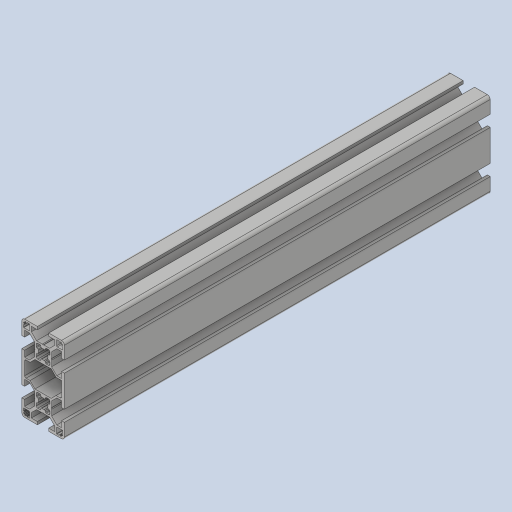
# Autodesk Inventor part: HFSLB6-3060-300
Saved by Autodesk Inventor 2023 (Build 270158000, 158)
## iProperties
Created: 2024-09-13
Part Number: HFSLB6-3060-300
Material: Generic
Catalog Web Link: www.cadenas.de
Description: NEFS6-3060, NEFSB6-3060, NEFSY6-3060, EFS6-3060, EFSB6-3060, HFS6-3060, HFSB6-3060, CAF6-3060, NFSL6-3060, HFSL6-3060, HFSLB6-3060, GFS6-3060, HFSY6-3060-Aluminum Frames -6 Series-2 Row Groove 30x60 mm Square-Specified Length
Vendor: MISUMI
Document SubType Name: Modeling
Designer: psAdmin
Manufacturer: MISUMI
Mass: 145.426 g
Surface Area: 1809.35 cm^2
Volume: 145.426 cm^3
Density: 1 g/cm^3
Appearance: PSOLRGB-175-175-175
Category: PARTsolutions
Company: MISUMI
PSOL_IDENT_0: {$CADENAS_DATA/23d-libs/misumi/metric/38_al_extrusions_blackets/6/hfs6_3060.prj},759 {VTYP=3D},{NB=H
PSOL_IDENT_1: FSLB6-3060-300},{LINA=HFSLB6-3060-300},{NN=NEFS6-3060, NEFSB6-3060, NEFSY6-3060, EFS6-3060, EFSB6-30
PSOL_IDENT_2: 60, HFS6-3060, HFSB6-3060, CAF6-3060, NFSL6-3060, HFSL6-3060, HFSLB6-3060, GFS6-3060, HFSY6-3060},{D
PSOL_IDENT_3: ATE=31.01.2024 10:05:17},{GEOMDATE=26.07.2023 02:49:00},{VERSION=},{LINEID=70},{WBVAR=L,ALT1,ALT2,AL
PSOL_IDENT_4: T3,ALT4,ALT5,CP5,DL5,DR5,ALT6,ALT9,ALT10,ALT11,DD6SE,DD6,HP6,NHL6,DL6,NHR6,DR6,ALT7,ALT8,NH9,AH,BH,C
PSOL_IDENT_5: H,DH,EH,NH10,AV,BV,CV,DV,EV,NH11,AP,BP,CP,DP,EP,ALT12,ALT13,Z,NH12,XA,XB,XC,XD,XE,NH13,YA,YB,YC,YD,Y
PSOL_IDENT_6: E,ALT14,HP14,DL14,DR14,ALT15,HP15,DL15,DR15,ALT16,HP16,DL16,DR16,ALT17,HQ17,JLP,ALT18,HQ18,KLP,ALT19
PSOL_IDENT_7: ,ALT20},{WBNUMERIC=L,DD6,NH9,AH,BH,CH,DH,EH,NH10,AV,BV,CV,DV,EV,NH11,AP,BP,CP,DP,EP,NH12,XA,XB,XC,XD
PSOL_IDENT_8: ,XE,NH13,YA,YB,YC,YD,YE,HQ17,JLP,HQ18,KLP}  {NB=HFSLB6-3060-300},{LINA=HFSLB6-3060-300},{KT=DUMMY},{
PSOL_IDENT_9: PN=HFSLB6-3060-300},{TPS=HFSLB6-3060},{MAT=A6N01SS-T5 Aluminum Alloy},{ST=Black Anodize},{FRMW=30},{
PSOL_IDENT_10: FRMH=60},{FRD=6.8},{L=300.0},{MASS=1.29},{SA=476},{LX=4.87x10^4},{LY=17.87x10^4},{ALT1=},{M1=0},{IDM
PSOL_IDENT_11: 1=6.647},{DALT1=4.2},{DPL1=0},{DPR1=0},{ALT1PN=},{ALT2=},{ALT2ALG= '','w/o End Tapping (Insert)','LH
PSOL_IDENT_12: P','with LHP (Tapping on the Left (Insert))','RHP','with RHP (Tapping on the Right (Insert))','HPW','
PSOL_IDENT_13: with HPW (Tapping on Both Ends (Insert))' },{M2=0},{DP2=0},{ALT2PN=},{ALT3=},{ALT3ALG= '','N/A' },{M
PSOL_IDENT_14: 3=0},{IDM3=4.134},{DP3=0},{ALT3PN=},{ALT4=},{ALT4ALG= '', 'w/o SC (High Precision Cut)', 'SC', 'with
PSOL_IDENT_15: SC (High Precision Cut)' },{ALT4PN=},{ALT5=},{ALT5ALG= '','w/o 45 Degree Cut','1','with 45 Degree C
PSOL_IDENT_16: ut' },{CP5=},{CP5ALG= '','N/A' },{DL5=},{DL5ALG= '','N/A' },{DR5=},{DR5ALG= '','N/A' },{FRMLALT5=0},
PSOL_IDENT_17: {FRMRALT5=0},{ALT5PN=},{ALT6=},{ALT6ALG= '','w/o Fastening Location Wrench Access Hole Alterations','
PSOL_IDENT_18: 1','with Fastening Location Wrench Access Hole Alterations' },{ALT9=},{ALT9ALG= '','w/o Location Spe
PSOL_IDENT_19: cified Wrench Access Hole Alteratons (Horizontal)','1','with Location Specified Wrench Access Hole A
PSOL_IDENT_20: lteratons (Horizontal)' },{ALT10=},{ALT10ALG= '','w/o Location Specified Wrench Access Hole Alterato
PSOL_IDENT_21: ns (Vertical)','1','with Location Specified Wrench Access Hole Alteratons (Vertical)' },{ALT11=},{AL
PSOL_IDENT_22: T11ALG= '','w/o Location Specified Wrench Access Hole Alteratons (Crisscross)','1','with Location Sp
PSOL_IDENT_23: ecified Wrench Access Hole Alteratons (Crisscross)' },{DD6SE=},{DD6SEALG= '','N/A' },{DD6=0},{DD6ALG=
PSOL_IDENT_24: 0},{HP6=},{HP6ALG= '','N/A' },{NHL6=},{NHL6ALG= '','N/A' },{DL6=},{DL6ALG= '','N/A' },{NHR6=},{NHR6A
PSOL_IDENT_25: LG= '','N/A' },{DR6=},{DR6ALG= '','N/A' },{DD6PN=},{HL6=0},{HL6D=0},{HR6=0},{HR6D=0},{J6=0},{J6D=0},
PSOL_IDENT_26: {K6=0},{K6D=0},{ALT7=},{ALT7ALG= '','N/A' },{ALT8=},{ALT8ALG= '','N/A' },{ALT678PN=},{NH9=0},{NH9MAX=
PSOL_IDENT_27: 5},{NH9ALG=[0]},{AH=0.0},{AHMIN=7},{AHMAX=295},{AHALG=[0]},{BH=0.0},{BHMIN=2},{BHMAX=297},{BHALG=[0]
PSOL_IDENT_28: },{CH=0.0},{CHMIN=2},{CHMAX=299},{CHALG=[0]},{DH=0.0},{DHMIN=2},{DHMAX=301},{DHALG=[0]},{EH=0.0},{EH
PSOL_IDENT_29: MIN=2},{EHMAX=293},{EHALG=[0]},{NH10=0},{NH10MAX=5},{NH10ALG=[0]},{AV=0.0},{AVMIN=7},{AVMAX=295},{AV
PSOL_IDENT_30: ALG=[0]},{BV=0.0},{BVMIN=2},{BVMAX=297},{BVALG=[0]},{CV=0.0},{CVMIN=2},{CVMAX=299},{CVALG=[0]},{DV=0
PSOL_IDENT_31: .0},{DVMIN=2},{DVMAX=301},{DVALG=[0]},{EV=0.0},{EVMIN=2},{EVMAX=293},{EVALG=[0]},{NH11=0},{NH11MAX=5
PSOL_IDENT_32: },{NH11ALG=[0]},{AP=0.0},{APMIN=7},{APMAX=295},{APALG=[0]},{BP=0.0},{BPMIN=2},{BPMAX=297},{BPALG=[0]
PSOL_IDENT_33: },{CP=0.0},{CPMIN=2},{CPMAX=299},{CPALG=[0]},{DP=0.0},{DPMIN=2},{DPMAX=301},{DPALG=[0]},{EP=0.0},{EP
PSOL_IDENT_34: MIN=2},{EPMAX=293},{EPALG=[0]},{ALT9PN=},{ALT10PN=},{ALT11PN=},{ALT91011PN=},{ALT12=},{ALT12ALG= '','
PSOL_IDENT_35: w/o Counterbore Hole in Specified Position (Vertical)','1','with Counterbore Hole in Specified Posit
PSOL_IDENT_36: ion (Vertical)' },{ALT13=},{ALT13ALG= '','w/o Counterbore Hole in Specified Position (Horizontal)','
PSOL_IDENT_37: 1','with Counterbore Hole in Specified Position (Horizontal)' },{Z=},{ZALG= '','N/A' },{DD12=0.0},{D
PSOL_IDENT_38: D112=0.0},{NH12=0},{NH12MAX=5},{NH12ALG=[0]},{XA=0.0},{XAMIN=7},{XAMAX=295},{XAALG=[0]},{XB=0.0},{XB
PSOL_IDENT_39: MIN=2},{XBMAX=297},{XBALG=[0]},{XC=0.0},{XCMIN=2},{XCMAX=299},{XCALG=[0]},{XD=0.0},{XDMIN=2},{XDMAX=
PSOL_IDENT_40: 301},{XDALG=[0]},{XE=0.0},{XEMIN=2},{XEMAX=293},{XEALG=[0]},{NH13=0},{NH13MAX=5},{NH13ALG=[0]},{YA=0
PSOL_IDENT_41: .0},{YAMIN=7},{YAMAX=295},{YAALG=[0]},{YB=0.0},{YBMIN=2},{YBMAX=297},{YBALG=[0]},{YC=0.0},{YCMIN=2},
PSOL_IDENT_42: {YCMAX=299},{YCALG=[0]},{YD=0.0},{YDMIN=2},{YDMAX=301},{YDALG=[0]},{YE=0.0},{YEMIN=2},{YEMAX=293},{Y
PSOL_IDENT_43: EALG=[0]},{ALT12PN=},{ALT13PN=},{ALT1213PN=},{ALT14=},{ALT14ALG= '','w/o D Type Hole Alteration','1'
PSOL_IDENT_44: ,'with D Type Hole Alteration' },{HP14=},{HP14ALG= '','N/A' },{DL14=},{DL14ALG= '','N/A' },{DR14=},{
PSOL_IDENT_45: DR14ALG= '','N/A' },{H14=0},{D14=0.0},{ALT14PN=},{ALT15=},{ALT15ALG= '','w/o S Type Hole Alteration'
PSOL_IDENT_46: ,'1','with S Type Hole Alteration' },{HP15=},{HP15ALG= '','N/A' },{DL15=},{DL15ALG= '','N/A' },{DR15=
PSOL_IDENT_47: },{DR15ALG= '','N/A' },{H15=0},{D115=0.0},{D215=0.0},{ALT15PN=},{ALT16=},{ALT16ALG= '','w/o M Type H
PSOL_IDENT_48: ole Alteration','1','with M Type Hole Alteration' },{HP16=},{HP16ALG= '','N/A' },{DL16=},{DL16ALG= ''
PSOL_IDENT_49: ,'N/A' },{DR16=},{DR16ALG= '','N/A' },{H116=0},{D16=0.0},{ALT16PN=},{ALT17=},{ALT17ALG= '','w/o L Ty
PSOL_IDENT_50: pe Hole Alteration (Top)','1','with L Type Hole Alteration (Top)' },{HQ17=0},{HQ17ALG=0},{JLP=0},{JL
PSOL_IDENT_51: PMIN=4.9},{JLPMAX=0},{JLPALG=[0]},{L17=0},{D17=0.0},{ALT18=},{ALT18ALG= '','w/o L Type Hole Alterati
PSOL_IDENT_52: on (Bottom)','1','with L Type Hole Alteration (Bottom)' },{HQ18=0},{HQ18ALG=0},{KLP=0},{KLPALG=[0]},
PSOL_IDENT_53: {KLPMIN=4.9},{KLPMAX=0},{L18=0},{D18=0.0},{ALT19=},{ALT19ALG= '','N/A' },{M19=0},{DP19=0},{ALT1718PN=
PSOL_IDENT_54: },{ALT19PN=},{ALT20=},{ALT20PN=},{ERRORALT01=OK},{ERRORALT02=OK},{ERRORALT03=OK},{ERRORALT05=OK},{ER
PSOL_IDENT_55: RORALT06091=OK},{ERRORALT06092=OK},{ERRORALT06093=OK},{ERRORALT06094=OK},{ERRORALT06101=OK},{ERRORAL
PSOL_IDENT_56: T06102=OK},{ERRORALT06103=OK},{ERRORALT06104=OK},{ERRORALT06111=OK},{ERRORALT06112=OK},{ERRORALT0611
PSOL_IDENT_57: 3=OK},{ERRORALT06114=OK},{ERRORALT06121=OK},{ERRORALT06122=OK},{ERRORALT06123=OK},{ERRORALT06124=OK}
PSOL_IDENT_58: ,{ERRORALT06131=OK},{ERRORALT06132=OK},{ERRORALT06133=OK},{ERRORALT06134=OK},{ERRORALT0614=OK},{ERRO
PSOL_IDENT_59: RALT0615=OK},{ERRORALT0616=OK},{ERRORALT06171=OK},{ERRORALT06172=OK},{ERRORALT06173=OK},{ERRORALT061
PSOL_IDENT_60: 81=OK},{ERRORALT06182=OK},{ERRORALT06183=OK},{ERRORALT0619=OK},{ERRORALT0911=OK},{ERRORALT0913=OK},{
PSOL_IDENT_61: ERRORALT0914=OK},{ERRORALT0915=OK},{ERRORALT0916=OK},{ERRORALT0917=OK},{ERRORALT0918=OK},{ERRORALT09
PSOL_IDENT_62: 19=OK},{ERRORALT1011=OK},{ERRORALT1012=OK},{ERRORALT1014=OK},{ERRORALT1015=OK},{ERRORALT1016=OK},{ER
PSOL_IDENT_63: RORALT1017=OK},{ERRORALT1018=OK},{ERRORALT1019=OK},{ERRORALT1112=OK},{ERRORALT1113=OK},{ERRORALT1114=
PSOL_IDENT_64: OK},{ERRORALT1115=OK},{ERRORALT1116=OK},{ERRORALT1117=OK},{ERRORALT1118=OK},{ERRORALT1119=OK},{ERROR
PSOL_IDENT_65: ALT1214=OK},{ERRORALT1215=OK},{ERRORALT1216=OK},{ERRORALT1217=OK},{ERRORALT1218=OK},{ERRORALT1219=OK
PSOL_IDENT_66: },{ERRORALT1314=OK},{ERRORALT1315=OK},{ERRORALT1316=OK},{ERRORALT1317=OK},{ERRORALT1318=OK},{ERRORAL
PSOL_IDENT_67: T1319=OK},{ERRORALT1415=OK},{ERRORALT1416=OK},{ERRORALT1417=OK},{ERRORALT1418=OK},{ERRORALT1419=OK},
PSOL_IDENT_68: {ERRORALT1516=OK},{ERRORALT1517=OK},{ERRORALT1518=OK},{ERRORALT1519=OK},{ERRORALT1617=OK},{ERRORALT1
PSOL_IDENT_69: 618=OK},{ERRORALT1619=OK},{ERRORALT1719=OK},{ERRORALT1819=OK},{ERRORPN=},{COLOR=}
NB: HFSLB6-3060-300
NN: NEFS6-3060, NEFSB6-3060, NEFSY6-3060, EFS6-3060, EFSB6-3060, HFS6-3060, HFSB6-3060, CAF6-3060, NFSL6-3060, HFSL6-3060, HFSLB6-3060, GFS6-3060, HFSY6-3060
NT: Aluminum Frames -6 Series-2 Row Groove 30x60 mm Square-Specified Length
NBSYN: $PN.
LINA: HFSLB6-3060-300
CATALOG: Misumi
PN: HFSLB6-3060-300
TPS: HFSLB6-3060
MAT: A6N01SS-T5 Aluminum Alloy
ST: Black Anodize
L: 300
MASS: 1.29
SA: 476
LX: 4.87x10^4
LY: 17.87x10^4
ALT1: w/o End Tapping
DPL1: 0
DPR1: 0
ALT2: w/o End Tapping (Insert)
M2: 0
DP2: 0
ALT3: N/A
M3: 0
DP3: 0
ALT4: w/o SC (High Precision Cut)
ALT5: w/o 45 Degree Cut
CP5: N/A
DL5: N/A
DR5: N/A
ALT6: w/o Fastening Location Wrench Access Hole Alterations
ALT9: w/o Location Specified Wrench Access Hole Alteratons (Horizontal)
ALT10: w/o Location Specified Wrench Access Hole Alteratons (Vertical)
ALT11: w/o Location Specified Wrench Access Hole Alteratons (Crisscross)
DD6SE: N/A
DD6: 0
HP6: N/A
NHL6: N/A
DL6: N/A
NHR6: N/A
DR6: N/A
HL6D: 0
HR6D: 0
J6D: 0
K6D: 0
ALT7: N/A
ALT8: N/A
NH9: 0
AH: 0
BH: 0
CH: 0
DH: 0
EH: 0
NH10: 0
AV: 0
BV: 0
CV: 0
DV: 0
EV: 0
NH11: 0
AP: 0
BP: 0
CP: 0
DP: 0
EP: 0
ALT12: w/o Counterbore Hole in Specified Position (Vertical)
ALT13: w/o Counterbore Hole in Specified Position (Horizontal)
Z: N/A
DD12: 0
DD112: 0
NH12: 0
XA: 0
XB: 0
XC: 0
XD: 0
XE: 0
NH13: 0
YA: 0
YB: 0
YC: 0
YD: 0
YE: 0
ALT14: w/o D Type Hole Alteration
HP14: N/A
DL14: N/A
DR14: N/A
H14: 0
D14: 0
ALT15: w/o S Type Hole Alteration
HP15: N/A
DL15: N/A
DR15: N/A
H15: 0
D115: 0
D215: 0
ALT16: w/o M Type Hole Alteration
HP16: N/A
DL16: N/A
DR16: N/A
H116: 0
D16: 0
ALT17: w/o L Type Hole Alteration (Top)
HQ17: 0
JLP: 0
D17: 0
ALT18: w/o L Type Hole Alteration (Bottom)
HQ18: 0
KLP: 0
D18: 0
ALT19: N/A
M19: 0
DP19: 0
ALT20: w/o CW (End Face C Chamfering)
SUPPLIER: MISUMI
ARTICLENO: HFSLB6-3060-300
BOMINFO: HFSLB6-3060-300
CREATOR: CADENAS GmbH
Title: HFSLB6-3060-300
Author: Cadenas PARTsolutions
Comments: Aluminum Frames -6 Series-2 Row Groove 30x60 mm Square-Specified Length
Autodesk Inventor part; units mm, degrees
sketch "Sketch_59" plane through (0, 0, 0) normal (0, 0, 1) x (1, 0, 0)
  line L0 (-15, -11) -> (-13, -11)
  line L1 (-13, -11) -> (-13, -6.75)
  line L2 (-13, -6.75) -> (-9.6642, -6.75)
  line L3 (-9.6642, -6.75) -> (-6, -10.4142)
  line L4 (-6, -10.4142) -> (-6, -14.4804)
  line L5 (-6, -14.4804) -> (-5.7, -15)
  line L6 (-5.7, -15) -> (-6, -15.5196)
  line L7 (-6, -15.5196) -> (-6, -19.5858)
  line L8 (-6, -19.5858) -> (-9.6642, -23.25)
  line L9 (-9.6642, -23.25) -> (-13, -23.25)
  line L10 (-13, -23.25) -> (-13, -19)
  line L11 (-13, -19) -> (-15, -19)
  line L12 (-15, -19) -> (-15, -28)
  arc A0 (-15, -28) -> (-13, -30) centre (-13, -28) ccw
  line L13 (-13, -30) -> (-4, -30)
  line L14 (-4, -30) -> (-4, -28)
  line L15 (-4, -28) -> (-8.25, -28)
  line L16 (-8.25, -28) -> (-8.25, -24.6642)
  line L17 (-8.25, -24.6642) -> (-4.5858, -21)
  line L18 (-4.5858, -21) -> (-0.5196, -21)
  line L19 (-0.5196, -21) -> (0, -20.7)
  line L20 (0, -20.7) -> (0.5196, -21)
  line L21 (0.5196, -21) -> (4.5858, -21)
  line L22 (4.5858, -21) -> (8.25, -24.6642)
  line L23 (8.25, -24.6642) -> (8.25, -28)
  line L24 (8.25, -28) -> (4, -28)
  line L25 (4, -28) -> (4, -30)
  line L26 (4, -30) -> (13, -30)
  arc A1 (13, -30) -> (15, -28) centre (13, -28) ccw
  line L27 (15, -28) -> (15, -19)
  line L28 (15, -19) -> (13, -19)
  line L29 (13, -19) -> (13, -23.25)
  line L30 (13, -23.25) -> (9.6642, -23.25)
  line L31 (9.6642, -23.25) -> (6, -19.5858)
  line L32 (6, -19.5858) -> (6, -15.5196)
  line L33 (6, -15.5196) -> (5.7, -15)
  line L34 (5.7, -15) -> (6, -14.4804)
  line L35 (6, -14.4804) -> (6, -10.4142)
  line L36 (6, -10.4142) -> (9.6642, -6.75)
  line L37 (9.6642, -6.75) -> (13, -6.75)
  line L38 (13, -6.75) -> (13, -11)
  line L39 (13, -11) -> (15, -11)
  line L40 (15, -11) -> (15, 11)
  line L41 (15, 11) -> (13, 11)
  line L42 (13, 11) -> (13, 6.75)
  line L43 (13, 6.75) -> (9.6642, 6.75)
  line L44 (9.6642, 6.75) -> (6, 10.4142)
  line L45 (6, 10.4142) -> (6, 14.4804)
  line L46 (6, 14.4804) -> (5.7, 15)
  line L47 (5.7, 15) -> (6, 15.5196)
  line L48 (6, 15.5196) -> (6, 19.5858)
  line L49 (6, 19.5858) -> (9.6642, 23.25)
  line L50 (9.6642, 23.25) -> (13, 23.25)
  line L51 (13, 23.25) -> (13, 19)
  line L52 (13, 19) -> (15, 19)
  line L53 (15, 19) -> (15, 28)
  arc A2 (15, 28) -> (13, 30) centre (13, 28) ccw
  line L54 (13, 30) -> (4, 30)
  line L55 (4, 30) -> (4, 28)
  line L56 (4, 28) -> (8.25, 28)
  line L57 (8.25, 28) -> (8.25, 24.6642)
  line L58 (8.25, 24.6642) -> (4.5858, 21)
  line L59 (4.5858, 21) -> (0.5196, 21)
  line L60 (0.5196, 21) -> (0, 20.7)
  line L61 (0, 20.7) -> (-0.5196, 21)
  line L62 (-0.5196, 21) -> (-4.5858, 21)
  line L63 (-4.5858, 21) -> (-8.25, 24.6642)
  line L64 (-8.25, 24.6642) -> (-8.25, 28)
  line L65 (-8.25, 28) -> (-4, 28)
  line L66 (-4, 28) -> (-4, 30)
  line L67 (-4, 30) -> (-13, 30)
  arc A3 (-13, 30) -> (-15, 28) centre (-13, 28) ccw
  line L68 (-15, 28) -> (-15, 19)
  line L69 (-15, 19) -> (-13, 19)
  line L70 (-13, 19) -> (-13, 23.25)
  line L71 (-13, 23.25) -> (-9.6642, 23.25)
  line L72 (-9.6642, 23.25) -> (-6, 19.5858)
  line L73 (-6, 19.5858) -> (-6, 15.5196)
  line L74 (-6, 15.5196) -> (-5.7, 15)
  line L75 (-5.7, 15) -> (-6, 14.4804)
  line L76 (-6, 14.4804) -> (-6, 10.4142)
  line L77 (-6, 10.4142) -> (-9.6642, 6.75)
  line L78 (-9.6642, 6.75) -> (-13, 6.75)
  line L79 (-13, 6.75) -> (-13, 11)
  line L80 (-13, 11) -> (-15, 11)
  line L81 (-15, 11) -> (-15, -11)
  line L82 (9.5, 28.6) -> (9.5, 25)
  arc A4 (9.5, 25) -> (10, 24.5) centre (10, 25) ccw
  line L83 (10, 24.5) -> (13.6, 24.5)
  arc A5 (13.6, 24.5) -> (13.8, 24.7) centre (13.6, 24.7) ccw
  line L84 (13.8, 24.7) -> (13.8, 26.2)
  arc A6 (13.8, 26.2) -> (13.6, 26.4) centre (13.6, 26.2) ccw
  line L85 (13.6, 26.4) -> (13.43, 26.4)
  arc A7 (13.23, 26.6) -> (13.43, 26.4) centre (13.43, 26.6) ccw
  line L86 (13.23, 26.6) -> (13.23, 27)
  arc A8 (13.43, 27.2) -> (13.23, 27) centre (13.43, 27) ccw
  line L87 (13.43, 27.2) -> (13.6, 27.2)
  arc A9 (13.6, 27.2) -> (13.8, 27.4) centre (13.6, 27.4) ccw
  line L88 (13.8, 27.4) -> (13.8, 27.6)
  arc A10 (13.8, 27.6) -> (13.5, 27.9) centre (13.5, 27.6) ccw
  line L89 (13.5, 27.9) -> (13.2, 27.9)
  arc A11 (12.9, 28.2) -> (13.2, 27.9) centre (13.2, 28.2) ccw
  line L90 (12.9, 28.2) -> (12.9, 28.5)
  arc A12 (12.9, 28.5) -> (12.6, 28.8) centre (12.6, 28.5) ccw
  line L91 (12.6, 28.8) -> (12.4, 28.8)
  arc A13 (12.4, 28.8) -> (12.2, 28.6) centre (12.4, 28.6) ccw
  line L92 (12.2, 28.6) -> (12.2, 28.43)
  arc A14 (12, 28.23) -> (12.2, 28.43) centre (12, 28.43) ccw
  line L93 (12, 28.23) -> (11.6, 28.23)
  arc A15 (11.4, 28.43) -> (11.6, 28.23) centre (11.6, 28.43) ccw
  line L94 (11.4, 28.43) -> (11.4, 28.6)
  arc A16 (11.4, 28.6) -> (11.2, 28.8) centre (11.2, 28.6) ccw
  line L95 (11.2, 28.8) -> (9.7, 28.8)
  arc A17 (9.7, 28.8) -> (9.5, 28.6) centre (9.7, 28.6) ccw
  arc A18 (9.5, -28.6) -> (9.7, -28.8) centre (9.7, -28.6) ccw
  line L96 (9.7, -28.8) -> (11.2, -28.8)
  arc A19 (11.2, -28.8) -> (11.4, -28.6) centre (11.2, -28.6) ccw
  line L97 (11.4, -28.6) -> (11.4, -28.43)
  arc A20 (11.6, -28.23) -> (11.4, -28.43) centre (11.6, -28.43) ccw
  line L98 (11.6, -28.23) -> (12, -28.23)
  arc A21 (12.2, -28.43) -> (12, -28.23) centre (12, -28.43) ccw
  line L99 (12.2, -28.43) -> (12.2, -28.6)
  arc A22 (12.2, -28.6) -> (12.4, -28.8) centre (12.4, -28.6) ccw
  line L100 (12.4, -28.8) -> (12.6, -28.8)
  arc A23 (12.6, -28.8) -> (12.9, -28.5) centre (12.6, -28.5) ccw
  line L101 (12.9, -28.5) -> (12.9, -28.2)
  arc A24 (13.2, -27.9) -> (12.9, -28.2) centre (13.2, -28.2) ccw
  line L102 (13.2, -27.9) -> (13.5, -27.9)
  arc A25 (13.5, -27.9) -> (13.8, -27.6) centre (13.5, -27.6) ccw
  line L103 (13.8, -27.6) -> (13.8, -27.4)
  arc A26 (13.8, -27.4) -> (13.6, -27.2) centre (13.6, -27.4) ccw
  line L104 (13.6, -27.2) -> (13.43, -27.2)
  arc A27 (13.23, -27) -> (13.43, -27.2) centre (13.43, -27) ccw
  line L105 (13.23, -27) -> (13.23, -26.6)
  arc A28 (13.43, -26.4) -> (13.23, -26.6) centre (13.43, -26.6) ccw
  line L106 (13.43, -26.4) -> (13.6, -26.4)
  arc A29 (13.6, -26.4) -> (13.8, -26.2) centre (13.6, -26.2) ccw
  line L107 (13.8, -26.2) -> (13.8, -24.7)
  arc A30 (13.8, -24.7) -> (13.6, -24.5) centre (13.6, -24.7) ccw
  line L108 (13.6, -24.5) -> (10, -24.5)
  arc A31 (10, -24.5) -> (9.5, -25) centre (10, -25) ccw
  line L109 (9.5, -25) -> (9.5, -28.6)
  arc A32 (-13, -4.55) -> (-12, -5.55) centre (-12, -4.55) ccw
  line L110 (-12, -5.55) -> (-9.1672, -5.55)
  line L111 (-9.1672, -5.55) -> (-5.7172, -9)
  line L112 (-5.7172, -9) -> (5.7172, -9)
  line L113 (5.7172, -9) -> (9.1672, -5.55)
  line L114 (9.1672, -5.55) -> (12, -5.55)
  arc A33 (12, -5.55) -> (13, -4.55) centre (12, -4.55) ccw
  line L115 (13, -4.55) -> (13, 5.55)
  line L116 (13, 5.55) -> (9.1672, 5.55)
  line L117 (9.1672, 5.55) -> (5.7172, 9)
  line L118 (5.7172, 9) -> (-5.7172, 9)
  line L119 (-5.7172, 9) -> (-9.1672, 5.55)
  line L120 (-9.1672, 5.55) -> (-12, 5.55)
  arc A34 (-12, 5.55) -> (-13, 4.55) centre (-12, 4.55) ccw
  line L121 (-13, 4.55) -> (-13, -4.55)
  line L122 (-13.8, -24.7) -> (-13.8, -26.2)
  arc A35 (-13.8, -26.2) -> (-13.6, -26.4) centre (-13.6, -26.2) ccw
  line L123 (-13.6, -26.4) -> (-13.43, -26.4)
  arc A36 (-13.23, -26.6) -> (-13.43, -26.4) centre (-13.43, -26.6) ccw
  line L124 (-13.23, -26.6) -> (-13.23, -27)
  arc A37 (-13.43, -27.2) -> (-13.23, -27) centre (-13.43, -27) ccw
  line L125 (-13.43, -27.2) -> (-13.6, -27.2)
  arc A38 (-13.6, -27.2) -> (-13.8, -27.4) centre (-13.6, -27.4) ccw
  line L126 (-13.8, -27.4) -> (-13.8, -27.6)
  arc A39 (-13.8, -27.6) -> (-13.5, -27.9) centre (-13.5, -27.6) ccw
  line L127 (-13.5, -27.9) -> (-13.2, -27.9)
  arc A40 (-12.9, -28.2) -> (-13.2, -27.9) centre (-13.2, -28.2) ccw
  line L128 (-12.9, -28.2) -> (-12.9, -28.5)
  arc A41 (-12.9, -28.5) -> (-12.6, -28.8) centre (-12.6, -28.5) ccw
  line L129 (-12.6, -28.8) -> (-12.4, -28.8)
  arc A42 (-12.4, -28.8) -> (-12.2, -28.6) centre (-12.4, -28.6) ccw
  line L130 (-12.2, -28.6) -> (-12.2, -28.43)
  arc A43 (-12, -28.23) -> (-12.2, -28.43) centre (-12, -28.43) ccw
  line L131 (-12, -28.23) -> (-11.6, -28.23)
  arc A44 (-11.4, -28.43) -> (-11.6, -28.23) centre (-11.6, -28.43) ccw
  line L132 (-11.4, -28.43) -> (-11.4, -28.6)
  arc A45 (-11.4, -28.6) -> (-11.2, -28.8) centre (-11.2, -28.6) ccw
  line L133 (-11.2, -28.8) -> (-9.7, -28.8)
  arc A46 (-9.7, -28.8) -> (-9.5, -28.6) centre (-9.7, -28.6) ccw
  line L134 (-9.5, -28.6) -> (-9.5, -25)
  arc A47 (-9.5, -25) -> (-10, -24.5) centre (-10, -25) ccw
  line L135 (-10, -24.5) -> (-13.6, -24.5)
  arc A48 (-13.6, -24.5) -> (-13.8, -24.7) centre (-13.6, -24.7) ccw
  line L136 (-13.8, 26.2) -> (-13.8, 24.7)
  arc A49 (-13.8, 24.7) -> (-13.6, 24.5) centre (-13.6, 24.7) ccw
  line L137 (-13.6, 24.5) -> (-10, 24.5)
  arc A50 (-10, 24.5) -> (-9.5, 25) centre (-10, 25) ccw
  line L138 (-9.5, 25) -> (-9.5, 28.6)
  arc A51 (-9.5, 28.6) -> (-9.7, 28.8) centre (-9.7, 28.6) ccw
  line L139 (-9.7, 28.8) -> (-11.2, 28.8)
  arc A52 (-11.2, 28.8) -> (-11.4, 28.6) centre (-11.2, 28.6) ccw
  line L140 (-11.4, 28.6) -> (-11.4, 28.43)
  arc A53 (-11.6, 28.23) -> (-11.4, 28.43) centre (-11.6, 28.43) ccw
  line L141 (-11.6, 28.23) -> (-12, 28.23)
  arc A54 (-12.2, 28.43) -> (-12, 28.23) centre (-12, 28.43) ccw
  line L142 (-12.2, 28.43) -> (-12.2, 28.6)
  arc A55 (-12.2, 28.6) -> (-12.4, 28.8) centre (-12.4, 28.6) ccw
  line L143 (-12.4, 28.8) -> (-12.6, 28.8)
  arc A56 (-12.6, 28.8) -> (-12.9, 28.5) centre (-12.6, 28.5) ccw
  line L144 (-12.9, 28.5) -> (-12.9, 28.2)
  arc A57 (-13.2, 27.9) -> (-12.9, 28.2) centre (-13.2, 28.2) ccw
  line L145 (-13.2, 27.9) -> (-13.5, 27.9)
  arc A58 (-13.5, 27.9) -> (-13.8, 27.6) centre (-13.5, 27.6) ccw
  line L146 (-13.8, 27.6) -> (-13.8, 27.4)
  arc A59 (-13.8, 27.4) -> (-13.6, 27.2) centre (-13.6, 27.4) ccw
  line L147 (-13.6, 27.2) -> (-13.43, 27.2)
  arc A60 (-13.23, 27) -> (-13.43, 27.2) centre (-13.43, 27) ccw
  line L148 (-13.23, 27) -> (-13.23, 26.6)
  arc A61 (-13.43, 26.4) -> (-13.23, 26.6) centre (-13.43, 26.6) ccw
  line L149 (-13.43, 26.4) -> (-13.6, 26.4)
  arc A62 (-13.6, 26.4) -> (-13.8, 26.2) centre (-13.6, 26.2) ccw
  constraints: 300 end point, 126 point on circle, 63 centre point
extrude "Extrusion1" add sketch "Sketch_59" against normal blind 300
sketch "Sketch_94" plane through (0, 0, 0) normal (0, 0, 1) x (1, 0, 0)
  line L0 (-4.8, 18.8) -> (-4.8, 17.2312)
  arc A0 (-4.8, 17.2312) -> (-4.4833, 16.766) centre (-4.3, 17.2312) ccw
  line L1 (-4.4833, 16.766) -> (-3.5987, 16.4176)
  arc A1 (-3.2971, 15.8303) -> (-3.5987, 16.4176) centre (-3.7819, 15.9524) ccw
  arc A2 (-3.2971, 15.8303) -> (-3.4, 15) centre (0, 15) ccw
  arc A3 (-3.4, 15) -> (-3.2971, 14.1697) centre (0, 15) ccw
  arc A4 (-3.5987, 13.5824) -> (-3.2971, 14.1697) centre (-3.7819, 14.0476) ccw
  line L2 (-3.5987, 13.5824) -> (-4.4833, 13.234)
  arc A5 (-4.4833, 13.234) -> (-4.8, 12.7688) centre (-4.3, 12.7688) ccw
  line L3 (-4.8, 12.7688) -> (-4.8, 11.2)
  arc A6 (-4.8, 11.2) -> (-3.8, 10.2) centre (-3.8, 11.2) ccw
  line L4 (-3.8, 10.2) -> (-2.2312, 10.2)
  arc A7 (-2.2312, 10.2) -> (-1.766, 10.5167) centre (-2.2312, 10.7) ccw
  line L5 (-1.766, 10.5167) -> (-1.4176, 11.4013)
  arc A8 (-0.8303, 11.7029) -> (-1.4176, 11.4013) centre (-0.9524, 11.2181) ccw
  arc A9 (-0.8303, 11.7029) -> (0, 11.6) centre (0, 15) ccw
  arc A10 (0, 11.6) -> (0.8303, 11.7029) centre (0, 15) ccw
  arc A11 (1.4176, 11.4013) -> (0.8303, 11.7029) centre (0.9524, 11.2181) ccw
  line L6 (1.4176, 11.4013) -> (1.766, 10.5167)
  arc A12 (1.766, 10.5167) -> (2.2312, 10.2) centre (2.2312, 10.7) ccw
  line L7 (2.2312, 10.2) -> (3.8, 10.2)
  arc A13 (3.8, 10.2) -> (4.8, 11.2) centre (3.8, 11.2) ccw
  line L8 (4.8, 11.2) -> (4.8, 12.7688)
  arc A14 (4.8, 12.7688) -> (4.4833, 13.234) centre (4.3, 12.7688) ccw
  line L9 (4.4833, 13.234) -> (3.5987, 13.5824)
  arc A15 (3.2971, 14.1697) -> (3.5987, 13.5824) centre (3.7819, 14.0476) ccw
  arc A16 (3.2971, 14.1697) -> (3.4, 15) centre (0, 15) ccw
  arc A17 (3.4, 15) -> (3.2971, 15.8303) centre (0, 15) ccw
  arc A18 (3.5987, 16.4176) -> (3.2971, 15.8303) centre (3.7819, 15.9524) ccw
  line L10 (3.5987, 16.4176) -> (4.4833, 16.766)
  arc A19 (4.4833, 16.766) -> (4.8, 17.2312) centre (4.3, 17.2312) ccw
  line L11 (4.8, 17.2312) -> (4.8, 18.8)
  arc A20 (4.8, 18.8) -> (3.8, 19.8) centre (3.8, 18.8) ccw
  line L12 (3.8, 19.8) -> (2.2312, 19.8)
  arc A21 (2.2312, 19.8) -> (1.766, 19.4833) centre (2.2312, 19.3) ccw
  line L13 (1.766, 19.4833) -> (1.4176, 18.5987)
  arc A22 (0.8303, 18.2971) -> (1.4176, 18.5987) centre (0.9524, 18.7819) ccw
  arc A23 (0.8303, 18.2971) -> (0, 18.4) centre (0, 15) ccw
  arc A24 (0, 18.4) -> (-0.8303, 18.2971) centre (0, 15) ccw
  arc A25 (-1.4176, 18.5987) -> (-0.8303, 18.2971) centre (-0.9524, 18.7819) ccw
  line L14 (-1.4176, 18.5987) -> (-1.766, 19.4833)
  arc A26 (-1.766, 19.4833) -> (-2.2312, 19.8) centre (-2.2312, 19.3) ccw
  line L15 (-2.2312, 19.8) -> (-3.8, 19.8)
  arc A27 (-3.8, 19.8) -> (-4.8, 18.8) centre (-3.8, 18.8) ccw
  constraints: 56 point on circle, 32 end point, 28 centre point
extrude "Extrusion2" cut sketch "Sketch_94" against normal blind 300
sketch "Sketch_113" plane through (0, 0, 0) normal (0, 0, 1) x (1, 0, 0)
  arc A0 (-4.8, -18.8) -> (-3.8, -19.8) centre (-3.8, -18.8) ccw
  line L0 (-3.8, -19.8) -> (-2.2312, -19.8)
  arc A1 (-2.2312, -19.8) -> (-1.766, -19.4833) centre (-2.2312, -19.3) ccw
  line L1 (-1.766, -19.4833) -> (-1.4176, -18.5987)
  arc A2 (-0.8303, -18.2971) -> (-1.4176, -18.5987) centre (-0.9524, -18.7819) ccw
  arc A3 (-0.8303, -18.2971) -> (0, -18.4) centre (0, -15) ccw
  arc A4 (0, -18.4) -> (0.8303, -18.2971) centre (0, -15) ccw
  arc A5 (1.4176, -18.5987) -> (0.8303, -18.2971) centre (0.9524, -18.7819) ccw
  line L2 (1.4176, -18.5987) -> (1.766, -19.4833)
  arc A6 (1.766, -19.4833) -> (2.2312, -19.8) centre (2.2312, -19.3) ccw
  line L3 (2.2312, -19.8) -> (3.8, -19.8)
  arc A7 (3.8, -19.8) -> (4.8, -18.8) centre (3.8, -18.8) ccw
  line L4 (4.8, -18.8) -> (4.8, -17.2312)
  arc A8 (4.8, -17.2312) -> (4.4833, -16.766) centre (4.3, -17.2312) ccw
  line L5 (4.4833, -16.766) -> (3.5987, -16.4176)
  arc A9 (3.2971, -15.8303) -> (3.5987, -16.4176) centre (3.7819, -15.9524) ccw
  arc A10 (3.2971, -15.8303) -> (3.4, -15) centre (0, -15) ccw
  arc A11 (3.4, -15) -> (3.2971, -14.1697) centre (0, -15) ccw
  arc A12 (3.5987, -13.5824) -> (3.2971, -14.1697) centre (3.7819, -14.0476) ccw
  line L6 (3.5987, -13.5824) -> (4.4833, -13.234)
  arc A13 (4.4833, -13.234) -> (4.8, -12.7688) centre (4.3, -12.7688) ccw
  line L7 (4.8, -12.7688) -> (4.8, -11.2)
  arc A14 (4.8, -11.2) -> (3.8, -10.2) centre (3.8, -11.2) ccw
  line L8 (3.8, -10.2) -> (2.2312, -10.2)
  arc A15 (2.2312, -10.2) -> (1.766, -10.5167) centre (2.2312, -10.7) ccw
  line L9 (1.766, -10.5167) -> (1.4176, -11.4013)
  arc A16 (0.8303, -11.7029) -> (1.4176, -11.4013) centre (0.9524, -11.2181) ccw
  arc A17 (0.8303, -11.7029) -> (0, -11.6) centre (0, -15) ccw
  arc A18 (0, -11.6) -> (-0.8303, -11.7029) centre (0, -15) ccw
  arc A19 (-1.4176, -11.4013) -> (-0.8303, -11.7029) centre (-0.9524, -11.2181) ccw
  line L10 (-1.4176, -11.4013) -> (-1.766, -10.5167)
  arc A20 (-1.766, -10.5167) -> (-2.2312, -10.2) centre (-2.2312, -10.7) ccw
  line L11 (-2.2312, -10.2) -> (-3.8, -10.2)
  arc A21 (-3.8, -10.2) -> (-4.8, -11.2) centre (-3.8, -11.2) ccw
  line L12 (-4.8, -11.2) -> (-4.8, -12.7688)
  arc A22 (-4.8, -12.7688) -> (-4.4833, -13.234) centre (-4.3, -12.7688) ccw
  line L13 (-4.4833, -13.234) -> (-3.5987, -13.5824)
  arc A23 (-3.2971, -14.1697) -> (-3.5987, -13.5824) centre (-3.7819, -14.0476) ccw
  arc A24 (-3.2971, -14.1697) -> (-3.4, -15) centre (0, -15) ccw
  arc A25 (-3.4, -15) -> (-3.2971, -15.8303) centre (0, -15) ccw
  arc A26 (-3.5987, -16.4176) -> (-3.2971, -15.8303) centre (-3.7819, -15.9524) ccw
  line L14 (-3.5987, -16.4176) -> (-4.4833, -16.766)
  arc A27 (-4.4833, -16.766) -> (-4.8, -17.2312) centre (-4.3, -17.2312) ccw
  line L15 (-4.8, -17.2312) -> (-4.8, -18.8)
  constraints: 56 point on circle, 32 end point, 28 centre point
extrude "Extrusion3" cut sketch "Sketch_113" against normal blind 300
ref_plane "CP_XY" through (0, 0, -150) normal (1, 0, 0) x (0, 0, -1)
ref_plane "CP_YZ" through (0, 0, -150) normal (0, 0, -1) x (0, 1, 0)
ref_plane "CP_ZX" through (0, 0, -150) normal (0, 1, 0) x (1, 0, 0)
ref_plane "to_frame_cap1_XY" through (0, 15, 0) normal (0, 0, 1) x (1, 0, 0)
ref_plane "to_frame_cap1_YZ" through (0, 15, 0) normal (1, 0, 0) x (0, 1, 0)
ref_plane "to_frame_cap1_ZX" through (0, 15, 0) normal (0, 1, 0) x (0, 0, 1)
ref_plane "to_frame_cap2_XY" through (0, 15, -300) normal (0, 0, -1) x (1, 0, 0)
ref_plane "to_frame_cap2_YZ" through (0, 15, -300) normal (1, 0, 0) x (0, -1, 0)
ref_plane "to_frame_cap2_ZX" through (0, 15, -300) normal (0, -1, 0) x (0, 0, -1)
body "Solid1"
